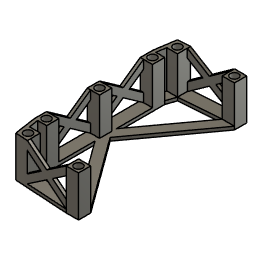
platform_hangfa-discovery-q2_stand-up-support (Autodesk Fusion 360 design; units mm, degrees)
Autodesk Fusion 360 part; units mm, degrees
note: some values were not read from the file. Set by a fixed rule: which sketch regions a step uses.
sketch "Sketch1" plane through (0, 0, 0) normal (0, 1, 0) x (1, 0, 0)
  circle A0 centre (0, 0) radius 5
  circle A1 centre (0, 65) radius 5
  circle A2 centre (0, 130) radius 5
  line L0 (0, 0) -> (4, 0)
  line L1 (4, 0) -> (4, -26.7021)
  line L2 (4, -26.7021) -> (0, -26.7021)
  line L3 (0, -26.7021) -> (0, 0)
  line L4 (4, -26.7021) -> (69.8787, -26.7021)
  line L5 (69.8787, -26.7021) -> (69.8787, -30.7021)
  line L6 (69.8787, -30.7021) -> (4, -30.7021)
  line L7 (4, -30.7021) -> (4, -26.7021)
  circle A3 centre (69.8787, -30.7021) radius 5
  circle A4 centre (4, -26.7021) radius 5
  line L8 (0, 130) -> (4, 130)
  line L9 (4, 130) -> (4, 156.7021)
  line L10 (4, 156.7021) -> (0, 156.7021)
  line L11 (0, 156.7021) -> (0, 130)
  circle A5 centre (4, 156.7021) radius 5
  line L12 (4, 156.7021) -> (69.8787, 156.7021)
  line L13 (69.8787, 156.7021) -> (69.8787, 160.7021)
  line L14 (69.8787, 160.7021) -> (4, 160.7021)
  line L15 (4, 160.7021) -> (4, 156.7021)
  circle A6 centre (69.8787, 160.7021) radius 5
  line L16 (11.5, 164.2021) -> (-3.5, 164.2021)
  line L17 (-3.5, 164.2021) -> (-3.5, 149.2021)
  line L18 (-3.5, 149.2021) -> (11.5, 149.2021)
  line L19 (11.5, 149.2021) -> (11.5, 164.2021)
  line L20 (11.5, 164.2021) -> (-3.5, 149.2021) construction
  line L21 (-3.5, 164.2021) -> (11.5, 149.2021) construction
  line L22 (77.3787, 168.2021) -> (62.3787, 168.2021)
  line L23 (62.3787, 168.2021) -> (62.3787, 153.2021)
  line L24 (62.3787, 153.2021) -> (77.3787, 153.2021)
  line L25 (77.3787, 153.2021) -> (77.3787, 168.2021)
  line L26 (77.3787, 168.2021) -> (62.3787, 153.2021) construction
  line L27 (62.3787, 168.2021) -> (77.3787, 153.2021) construction
  line L28 (-7.5, 122.5) -> (7.5, 122.5)
  line L29 (7.5, 122.5) -> (7.5, 137.5)
  line L30 (7.5, 137.5) -> (-7.5, 137.5)
  line L31 (-7.5, 137.5) -> (-7.5, 122.5)
  line L32 (-7.5, 122.5) -> (7.5, 137.5) construction
  line L33 (7.5, 122.5) -> (-7.5, 137.5) construction
  line L34 (-7.5, 72.5) -> (7.5, 72.5)
  line L35 (7.5, 72.5) -> (7.5, 57.5)
  line L36 (7.5, 57.5) -> (-7.5, 57.5)
  line L37 (-7.5, 57.5) -> (-7.5, 72.5)
  line L38 (-7.5, 72.5) -> (7.5, 57.5) construction
  line L39 (7.5, 72.5) -> (-7.5, 57.5) construction
  line L40 (-7.5, 7.5) -> (7.5, 7.5)
  line L41 (7.5, 7.5) -> (7.5, -7.5)
  line L42 (7.5, -7.5) -> (-7.5, -7.5)
  line L43 (-7.5, -7.5) -> (-7.5, 7.5)
  line L44 (-7.5, 7.5) -> (7.5, -7.5) construction
  line L45 (7.5, 7.5) -> (-7.5, -7.5) construction
  line L46 (-3.5, -34.2021) -> (11.5, -34.2021)
  line L47 (11.5, -34.2021) -> (11.5, -19.2021)
  line L48 (11.5, -19.2021) -> (-3.5, -19.2021)
  line L49 (-3.5, -19.2021) -> (-3.5, -34.2021)
  line L50 (-3.5, -34.2021) -> (11.5, -19.2021) construction
  line L51 (11.5, -34.2021) -> (-3.5, -19.2021) construction
  line L52 (77.3787, -23.2021) -> (62.3787, -23.2021)
  line L53 (62.3787, -23.2021) -> (62.3787, -38.2021)
  line L54 (62.3787, -38.2021) -> (77.3787, -38.2021)
  line L55 (77.3787, -38.2021) -> (77.3787, -23.2021)
  line L56 (77.3787, -23.2021) -> (62.3787, -38.2021) construction
  line L57 (62.3787, -23.2021) -> (77.3787, -38.2021) construction
  line L58 (-7.5, 7.5) -> (-7.5, 57.5)
  line L59 (7.5, 57.5) -> (7.5, 7.5)
  line L60 (-7.5, -7.5) -> (-3.5, -34.2021)
  line L61 (7.5, -7.5) -> (11.5, -19.2021)
  line L62 (11.5, -19.2021) -> (62.3787, -23.2021)
  line L63 (-3.5, -34.2021) -> (62.3787, -38.2021)
  line L64 (-7.5, 137.5) -> (-3.5, 164.2021)
  line L65 (7.5, 137.5) -> (11.5, 149.2021)
  line L66 (11.5, 149.2021) -> (62.3787, 153.2021)
  line L67 (-3.5, 164.2021) -> (62.3787, 168.2021)
  line L68 (-7.5, 122.5) -> (-7.5, 72.5)
  line L69 (7.5, 72.5) -> (7.5, 122.5)
  line L70 (62.3787, 168.2021) -> (-7.5, 72.5)
  line L71 (77.3787, 153.2021) -> (7.5, 57.5)
  line L72 (-7.5, 57.5) -> (62.3787, -38.2021)
  line L73 (7.5, 72.5) -> (77.3787, -23.2021)
  line L74 (62.3787, 153.2021) -> (72.1625, 146.0582)
  line L75 (62.3787, -23.2021) -> (72.1625, -16.0582)
  line L76 (7.5, 57.5) -> (-2.2838, 50.3562)
  line L77 (7.5, 57.5) -> (14.6438, 62.7162)
  line L78 (7.5, 72.5) -> (14.6438, 67.2838)
  line L79 (7.5, 72.5) -> (-2.2838, 79.6438)
  line L80 (62.3787, 153.2021) -> (4.86, 74.4276)
  line L81 (62.3787, -23.2021) -> (4.86, 55.5724)
  line L82 (11.5, -34.2021) -> (11.5, -35.1128)
  line L83 (11.5, 164.2021) -> (11.5, 165.1128)
  line L84 (-3.5, -19.2021) -> (-5.747, -19.2021)
  line L85 (-3.5, 149.2021) -> (-5.747, 149.2021)
  point P0 (4, 156.7021)
  point P1 (69.8787, 160.7021)
  point P2 (0, 130)
  point P3 (0, 65)
  point P4 (4, -26.7021)
  point P5 (69.8787, -30.7021)
  dimension "d1" = 10
  dimension "d4" = 0
  dimension "d5" = 65
  dimension "d6" = 4
  dimension "d7" = 26.7021
  dimension "d8" = 65.8787
  dimension "d9" = 4
  dimension "d10" = 10
  dimension "d11" = 10
  dimension "d12" = 4
  dimension "d13" = 26.7021
  dimension "d14" = 10
  dimension "d15" = 65.8787
  dimension "d16" = 4
  dimension "d17" = 10
  dimension "d18" = 15
  dimension "d19" = 15
  dimension "d20" = 15
  dimension "d21" = 15
  dimension "d22" = 15
  dimension "d23" = 15
  dimension "d24" = 15
  dimension "d25" = 15
  dimension "d26" = 15
  dimension "d27" = 15
  dimension "d28" = 15
  dimension "d29" = 15
  dimension "d30" = 15
  dimension "d31" = 15
  constraint coincident A0.centre L0.start
  constraint horizontal L0
  constraint vertical L1
  constraint horizontal L2
  constraint vertical L3
  constraint horizontal L4
  constraint vertical L5
  constraint horizontal L6
  constraint vertical L7
  constraint coincident P5 L5.end
  constraint coincident P4 L1.end
  constraint horizontal L8
  constraint vertical L9
  constraint horizontal L10
  constraint vertical L11
  constraint coincident P2 A2.centre
  constraint coincident P0 L9.end
  constraint horizontal L12
  constraint vertical L13
  constraint horizontal L14
  constraint vertical L15
  constraint coincident P1 L13.end
  constraint horizontal L16
  constraint perpendicular L16 L17
  constraint parallel L16 L18
  constraint parallel L17 L19
  constraint coincident L20 P0
  constraint coincident L21 P0
  constraint horizontal L22
  constraint perpendicular L22 L23
  constraint parallel L22 L24
  constraint parallel L23 L25
  constraint coincident L26 P1
  constraint coincident L27 P1
  constraint horizontal L28
  constraint perpendicular L28 L29
  constraint parallel L28 L30
  constraint parallel L29 L31
  constraint coincident L32 P2
  constraint coincident L33 P2
  constraint horizontal L34
  constraint perpendicular L34 L35
  constraint parallel L34 L36
  constraint parallel L35 L37
  constraint coincident L38 P3
  constraint coincident L39 P3
  constraint coincident P3 A1.centre
  constraint horizontal L40
  constraint perpendicular L40 L41
  constraint parallel L40 L42
  constraint parallel L41 L43
  constraint coincident L44 A0.centre
  constraint coincident L45 A0.centre
  constraint horizontal L46
  constraint perpendicular L46 L47
  constraint parallel L46 L48
  constraint parallel L47 L49
  constraint coincident L50 P4
  constraint coincident L51 P4
  constraint horizontal L52
  constraint perpendicular L52 L53
  constraint parallel L52 L54
  constraint parallel L53 L55
  constraint coincident L56 P5
  constraint coincident L57 P5
  constraint coincident L71 L74.end
  constraint perpendicular L71 L74
  constraint coincident L73 L75.end
  constraint perpendicular L73 L75
  constraint coincident L72 L76.end
  constraint perpendicular L72 L76
  constraint coincident L73 L77.end
  constraint perpendicular L73 L77
  constraint coincident L71 L78.end
  constraint perpendicular L71 L78
  constraint coincident L70 L79.end
  constraint perpendicular L70 L79
  constraint coincident L79 L80.end
  constraint perpendicular L79 L80
  constraint coincident L76 L81.end
  constraint perpendicular L76 L81
  constraint coincident L63 L82.end
  constraint perpendicular L46 L82
  constraint coincident L67 L83.end
  constraint perpendicular L16 L83
  constraint coincident L60 L84.end
  constraint perpendicular L49 L84
  constraint coincident L64 L85.end
  constraint perpendicular L17 L85
  measures "d1" diameter of A0
  measures "d6" distance of A0.centre L0.end
  measures "d7" distance of A0.centre L2.end
  measures "d8" distance of P4 L4.end
  measures "d9" distance of P4 L6.end
  measures "d10" diameter of A3
  measures "d11" diameter of A4
  measures "d12" distance of P2 L8.end
  measures "d13" distance of P2 L10.end
  measures "d14" diameter of A5
  measures "d15" distance of P0 L12.end
  measures "d16" distance of P0 L14.end
  measures "d17" diameter of A6
  measures "d18" distance of L17.end L18.end
  measures "d19" distance of L16.end L17.end
  measures "d20" distance of L23.end L24.end
  measures "d21" distance of L22.end L23.end
  measures "d22" distance of L29.end L30.end
  measures "d23" distance of L28.end L29.end
  measures "d24" distance of L35.end L36.end
  measures "d25" distance of L34.end L35.end
  measures "d26" distance of L41.end L42.end
  measures "d27" distance of L40.end L41.end
  measures "d28" distance of L47.end L48.end
  measures "d29" distance of L46.end L47.end
  measures "d30" distance of L53.end L54.end
  measures "d31" distance of L52.end L53.end
extrude "Extrude1" add sketch "Sketch1" along normal blind 50 contours A0 L1 L3 L40 L41 L42 L43 | A0 L1 L3 L42 | L1 L3 A4 L48 | L3 L6 A4 L46 L47 L48 L49 | L1 L4 A4 L47 L48 | L49 L60 L84 | L4 L6 A4 L47 | L46 L63 L82 | L34 L35 L36 L37 | L4 L6 A3 L52 L53 L54 L55 | A2 L9 L11 L28 L29 L30 L31 | L4 L6 A3 L53 | L12 L14 A6 L22 L23 L24 L25 | A2 L9 L11 L30 | L17 L64 L85 | L12 L14 A6 L23 | L9 A5 L12 L18 L19 | L11 A5 L14 L16 L17 L18 L19 | L9 L11 A5 L18 | L16 L67 L83 | A5 L12 L14 L19 makes body 1 at (8.9752, 16.6667, -157.1999) makes body 2 at (8.9938, 33.3333, 26.9513) makes body 3 at (4.9752, 16.6667, -64.5022) makes body 4 at (4.9752, 16.6667, -130.4978) makes body 5 at (74.8538, 16.6667, 30.2042) makes body 6 at (4.9938, 33.3333, 0.2492) makes body 7 at (65.2713, 33.3333, -158.7599)
extrude "Extrude2" add sketch "Sketch1" along normal blind 4 separate body contours L1 L3 L42 L48 | L3 L42 L48 L60 L84 | L1 L42 L48 L61 | L49 L60 L84 | L40 L58 L59 L72 | L4 L47 L62 L72 | L46 L63 L82 | L36 L72 L76 | L4 L6 L47 L72 | L4 L53 L62 L72 | L59 L72 L76 L81 | L6 L47 L63 L72 L82 | L59 L73 L75 L77 L81 | L35 L71 L73 | L59 L76 L81 | L71 L73 L77 | L34 L70 L79 | L28 L68 L69 L70 | L4 L6 L53 L72 | L52 L73 L75 | L6 L53 L72 | L69 L79 L80 | L71 L73 L78 | L69 L71 L74 L78 L80 | L69 L70 L79 L80 | L11 L18 L30 L64 L85 | L12 L23 L66 L70 | L24 L71 L74 | L9 L18 L30 L65 | L9 L11 L18 L30 | L17 L64 L85 | L12 L19 L66 L70 | L12 L14 L23 L70 | L16 L67 L83 | L12 L14 L19 L70 | L14 L23 L70 | L14 L19 L67 L70 L83 makes body 8 at (-2.5, 0, -91.0144)
combine "Combine1" operation add target body 8 tool bodies 7 6 5 4 3 2 1
extrude "Extrude3" add sketch "Sketch1" along normal blind 40 contours A0 L0 L1 L3 | A0 L0 L1 L3 | L1 L2 L3 A4 | L2 L3 L6 L7 A4 | L1 L4 A4 | L4 L6 L7 A4 | L4 L5 L6 A3 | L4 L5 L6 A3 | A2 L8 L9 L11 | A2 L8 L9 L11 | L12 L13 L14 A6 | L12 L13 L14 A6 | L10 L11 A5 L14 L15 | L9 L10 L11 A5 | L9 A5 L12 | A5 L12 L14 L15 | A1 bodies 8
sketch "Sketch2" plane through (-7.5, 0, 0) normal (-1, 0, 0) x (0, 0, 1)
  line L0 (-137.5, 0) -> (7.5, 0)
  line L1 (7.5, 0) -> (7.5, 4)
  line L2 (7.5, 4) -> (7.5, 50)
  line L3 (7.5, 50) -> (-7.5, 50)
  line L4 (-7.5, 50) -> (-7.5, 4)
  line L5 (-7.5, 4) -> (-57.5, 4)
  line L6 (-57.5, 4) -> (-57.5, 50)
  line L7 (-57.5, 50) -> (-72.5, 50)
  line L8 (-72.5, 50) -> (-72.5, 4)
  line L9 (-72.5, 4) -> (-122.5, 4)
  line L10 (-122.5, 4) -> (-122.5, 50)
  line L11 (-122.5, 50) -> (-137.5, 50)
  line L12 (-137.5, 50) -> (-137.5, 4)
  line L13 (-137.5, 4) -> (-137.5, 0)
  line L14 (-122.5, 50) -> (-57.5, 4)
  line L15 (-137.5, 50) -> (-72.5, 4)
  line L16 (-72.5, 50) -> (-7.5, 4)
  line L17 (7.5, 4) -> (-57.5, 50)
  line L18 (7.5, 50) -> (-57.5, 4)
  line L19 (-7.5, 50) -> (-72.5, 4)
  line L20 (-57.5, 50) -> (-122.5, 4)
  line L21 (-72.5, 50) -> (-137.5, 4)
  constraint coincident L10.end L11.start
  constraint coincident L5.end L6.start
  constraint coincident L11.end L12.start
  constraint coincident L8.end L9.start
  constraint coincident L7.end L8.start
  constraint coincident L4.end L5.start
  constraint coincident L1.end L2.start
  constraint coincident L6.end L7.start
  constraint coincident L2.end L3.start
  constraint coincident L3.end L4.start
  constraint coincident L9.end L10.start
  constraint coincident L12.end L13.start
extrude "Extrude4" add sketch "Sketch2" against normal blind 4 contours L10 L15 L20 L21 | L4 L16 L17 L18 | L10 L14 L15 L21 | L14 L15 L20 L21 | L4 L17 L18 L19 | L16 L17 L18 L19 | L8 L14 L20 L21 | L8 L14 L15 L20 | L6 L16 L17 L19 | L6 L16 L18 L19 bodies 8
sketch "Sketch6" plane through (-2.0819, 0, 34.2882) normal (-0.060606, 0, 0.998162) x (0.998162, 0, 0.060606)
  line L0 (-1.4207, 0) -> (64.5793, 0)
  line L1 (64.5793, 0) -> (64.5793, 4)
  line L2 (64.5793, 4) -> (13.6069, 4)
  line L3 (13.6069, 4) -> (13.6069, 50)
  line L4 (13.6069, 50) -> (-1.4207, 50)
  line L5 (-1.4207, 50) -> (-1.4207, 0)
  line L6 (64.5793, 4) -> (64.5793, 50)
  line L7 (-1.4207, 4) -> (64.5793, 50)
  line L8 (13.6069, 4) -> (79.6069, 50)
  line L9 (64.5793, 4) -> (-1.4207, 50)
  line L10 (13.6069, 50) -> (79.6069, 4)
  line L11 (13.6069, 50) -> (11.6069, 50)
  line L12 (11.6069, 50) -> (11.6069, 40.9201)
  dimension "d41" = 46
  dimension "d44" = 2
  constraint coincident L1.end L2.start
  constraint perpendicular L2 L6
  constraint coincident L5 L7.start
  constraint coincident L2.end L3.start
  constraint parallel L7 L8
  constraint coincident L4.end L5.start
  constraint coincident L3.end L4.start
  constraint parallel L9 L10
  constraint perpendicular L3 L11
  constraint coincident L9 L12.end
  constraint perpendicular L11 L12
  measures "d41" distance of L1.end L6.end
  measures "d44" distance of L3.end L11.end
extrude "Extrude5" add sketch "Sketch6" against normal blind 4 contours L6 L8 L9 L10 | L3 L7 L8 L9 | L7 L8 L9 L10 | L3 L7 L9 L10 | L6 L7 L8 L10 bodies 8
extrude "Extrude6" add 1 faces at (11.5808, 43.0175, 33.7819) along direction (-0.998162, 0, -0.060606) blind 1 on bodies 8 bodies 8
extrude "Extrude7" add 1 faces at (11.6616, 10.9825, 32.4511) along direction (-0.998162, 0, -0.060606) blind 1 on bodies 8 bodies 8
sketch "Sketch7" plane through (-9.9462, 0, -163.8107) normal (-0.060606, 0, -0.998162) x (-0.998162, 0, 0.060606)
  line L0 (-21.4857, 4) -> (-72.4581, 4)
  line L1 (-72.4581, 4) -> (-72.4581, 0)
  line L2 (-72.4581, 0) -> (-6.4581, 0)
  line L3 (-6.4581, 0) -> (-6.4581, 50)
  line L4 (-6.4581, 50) -> (-21.4857, 50)
  line L5 (-21.4857, 50) -> (-21.4857, 4)
  line L6 (-72.4581, 4) -> (-6.4581, 50)
  line L7 (-21.4857, 50) -> (-87.4857, 4)
  line L8 (-72.4581, 4) -> (-72.4581, 50)
  line L9 (-72.4581, 50) -> (-6.4581, 4)
  line L10 (-21.4857, 4) -> (-87.4857, 50)
  dimension "d49" = 46
  constraint coincident L0.end L1.start
  constraint coincident L3.end L4.start
  constraint coincident L4.end L5.start
  constraint parallel L6 L7
  constraint perpendicular L0 L8
  constraint coincident L3 L9.end
  constraint coincident L0.start L5.end
  constraint parallel L9 L10
  measures "d49" distance of L0.end L8.end
extrude "Extrude8" add sketch "Sketch7" against normal blind 4 contours L5 L6 L9 L10 | L6 L7 L8 L10 | L6 L7 L9 L10 | L5 L6 L7 L9 | L7 L8 L9 L10 bodies 8
extrude "Extrude9" add 1 faces at (11.5808, 46.5087, -163.7819) along direction (-0.998162, 0, 0.060606) blind 1 on bodies 8 bodies 8
sketch "Sketch9" plane through (0, 4, 0) normal (0, 1, 0) x (-1, 0, 0)
  line L0 (-11.5, -149.2021) -> (5.747, -149.2021)
  line L1 (5.747, -149.2021) -> (7.5, -137.5)
  line L2 (7.5, -137.5) -> (-7.5, -137.5)
  line L3 (-7.5, -137.5) -> (-11.5, -149.2021)
  line L4 (-4.6401, -141.5) -> (-5.9055, -145.2021)
  line L5 (-5.9055, -145.2021) -> (2.3016, -145.2021)
  line L6 (2.3016, -145.2021) -> (2.8562, -141.5)
  line L7 (2.8562, -141.5) -> (-4.6401, -141.5)
  line L8 (2.8562, -141.5) -> (3.4554, -137.5)
  line L9 (2.3016, -145.2021) -> (1.7024, -149.2021)
  dimension "d54" = -4
  constraint coincident L2 L8.end
  constraint parallel L6 L8
  constraint coincident L0 L9.end
  constraint parallel L6 L9
  measures "d54" distance of L3
extrude "Extrude11" add sketch "Sketch9" along normal up to surface (46 mm away) contours L0 L1 L2 L6 L8 L9 bodies 8
sketch "Sketch10" plane through (0, 4, 0) normal (0, 1, 0) x (-1, 0, 0)
  line L0 (5.747, 19.2021) -> (-11.5, 19.2021)
  line L1 (-11.5, 19.2021) -> (-7.5, 7.5)
  line L2 (-7.5, 7.5) -> (7.5, 7.5)
  line L3 (7.5, 7.5) -> (5.747, 19.2021)
  line L4 (-5.9055, 15.2021) -> (-4.6401, 11.5)
  line L5 (-4.6401, 11.5) -> (2.8562, 11.5)
  line L6 (2.8562, 11.5) -> (2.3016, 15.2021)
  line L7 (2.3016, 15.2021) -> (-5.9055, 15.2021)
  line L8 (2.3016, 15.2021) -> (1.7024, 19.2021)
  line L9 (2.8562, 11.5) -> (3.4554, 7.5)
  dimension "d59" = -4
  constraint coincident L0 L8.end
  constraint parallel L6 L8
  constraint coincident L2 L9.end
  constraint parallel L6 L9
  measures "d59" distance of L1
extrude "Extrude12" add sketch "Sketch10" along normal up to surface (46 mm away) contours L0 L2 L3 L6 L8 L9 bodies 8
sketch "Sketch11" plane through (-27.481, 0, -4.1167) normal (-0.988965, 0, -0.148148) x (-0.148148, 0, 0.988965)
  line L0 (-161.8716, 0) -> (-134.8716, 0)
  line L1 (-134.8716, 0) -> (-134.8716, 50)
  line L2 (-134.8716, 50) -> (-161.8716, 50)
  line L3 (-161.8716, 50) -> (-161.8716, 0)
  line L4 (-123.3716, 11.5) -> (-123.3716, 38.5) construction
  line L5 (-123.3716, 38.5) -> (-173.3716, 38.5) construction
  line L6 (-173.3716, 38.5) -> (-173.3716, 11.5) construction
  line L7 (-173.3716, 11.5) -> (-123.3716, 11.5) construction
  dimension "d62" = 10
  text T0 "ADAM" font "Arial" height 10 align centre middle in box 27 x 50 at (-123.3716, 11.5) x (0, 1) y (-1, 0) spacing 1
extrude "Extrude13" cut sketch "Sketch11" against normal blind 1 text T0 bodies 8
sketch "Sketch12" plane through (-8.4342, 0, 1.2635) normal (-0.988965, 0, 0.148148) x (0.148148, 0, 0.988965)
  line L0 (6.3061, 50) -> (6.3061, 0)
  line L1 (6.3061, 0) -> (33.3061, 0)
  line L2 (33.3061, 0) -> (33.3061, 50)
  line L3 (33.3061, 50) -> (6.3061, 50)
  line L4 (44.8061, 11.5) -> (44.8061, 38.5) construction
  line L5 (44.8061, 38.5) -> (-5.1939, 38.5) construction
  line L6 (-5.1939, 38.5) -> (-5.1939, 11.5) construction
  line L7 (-5.1939, 11.5) -> (44.8061, 11.5) construction
  dimension "d65" = 10
  text T0 "ADAM" font "Arial" height 10 align centre middle in box 27 x 50 at (44.8061, 11.5) x (0, 1) y (-1, 0) spacing 1
extrude "Extrude14" cut sketch "Sketch12" against normal blind 1 text T0 bodies 8
equation "d7 = ( sqrt(27 * 27 - 4 * 4) ) * 1 mm"
equation "d8 = ( sqrt(66 * 66 - 4 * 4) ) * 1 mm"
equation "d13 = ( sqrt(27 * 27 - 4 * 4) ) * 1 mm"
equation "d15 = ( sqrt(66 * 66 - 4 * 4) ) * 1 mm"
equation "d41 = 50 mm - 4 mm"
equation "d49 = 50 mm - 4 mm"
